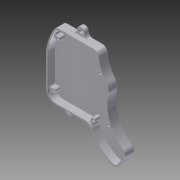
# Autodesk Inventor part: 20keyCaseRIght
Saved by Autodesk Inventor 2015 SP2 (Build 190223200, 223)
## iProperties
Created: 2015-12-14
Part Number: 20keyCaseRIght
Material: Aluminum 6061
Document SubType Name: Modeling
Designer: Josh
Density: 2.7 g/cm^3
Appearance: Aluminum - Flat
Author: Josh
Autodesk Inventor part; units mm, degrees
ref_plane "YZ Plane" through (0, 0, 0) normal (1, 0, 0) x (0, 1, 0)
ref_plane "XZ Plane" through (0, 0, 0) normal (0, 1, 0) x (-1, 0, 0)
ref_plane "XY Plane" through (0, 0, 0) normal (0, 0, 1) x (1, 0, 0)
sketch "Sketch1" plane through (0, 0, 0) normal (0, 0, 1) x (1, 0, 0)
  arc A0 (-34.3306, 52.1789) -> (-46.6208, 17.6368) centre (46.1813, 4.0752) ccw projected
  arc A1 (-46.6913, -8.336) -> (-46.6875, -8.1163) centre (-53.0375, -8.1163) ccw projected
  arc A2 (-46.6208, 17.6368) -> (-46.6875, 16.7186) centre (-40.3375, 16.7186) ccw projected
  arc A3 (-28.8795, 55.272) -> (-34.3306, 52.1789) centre (-28.8795, 48.922) ccw projected
  line L0 (-28.8795, 55.272) -> (26.3659, 55.272) projected
  arc A4 (32.6845, 49.5522) -> (26.3659, 55.272) centre (26.3659, 48.922) ccw projected
  arc A5 (32.6845, 49.5522) -> (45.4912, 18.6994) centre (90.0314, 55.272) ccw projected
  arc A6 (48.0197, 7.6526) -> (45.4912, 18.6994) centre (35.6761, 10.6401) ccw projected
  arc A7 (48.0197, 7.6526) -> (72.5516, -61.5815) centre (113.3553, -8.1601) ccw projected
  arc A8 (74.0573, -70.0323) -> (72.5516, -61.5815) centre (68.6971, -66.6278) ccw projected
  line L1 (65.6044, -83.341) -> (74.0573, -70.0323) projected
  arc A9 (58.0785, -85.9058) -> (65.6044, -83.341) centre (60.2442, -79.9365) ccw projected
  arc A10 (25.4201, -55.2506) -> (58.0785, -85.9058) centre (77.431, -32.5649) ccw projected
  arc A11 (25.4201, -55.2506) -> (13.7792, -47.628) centre (13.7792, -60.328) ccw projected
  arc A12 (-49.8625, -34.928) -> (-33.9875, -50.803) centre (-33.9875, -34.928) ccw
  arc A13 (-37.0562, 53.8074) -> (-49.7624, 18.0959) centre (46.1813, 4.0752) ccw
  arc A14 (-28.8795, 58.447) -> (-37.0562, 53.8074) centre (-28.8795, 48.922) ccw
  arc A15 (35.8439, 49.8674) -> (26.3659, 58.447) centre (26.3659, 48.922) ccw
  arc A16 (35.8439, 49.8674) -> (47.945, 20.7143) centre (90.0314, 55.272) ccw
  arc A17 (51.1056, 6.9058) -> (47.945, 20.7143) centre (35.6761, 10.6401) ccw
  arc A18 (51.1056, 6.9058) -> (74.4788, -59.0583) centre (113.3553, -8.1601) ccw
  arc A19 (76.7374, -71.7346) -> (74.4788, -59.0583) centre (68.6971, -66.6278) ccw
  arc A20 (22.5099, -56.5199) -> (13.7792, -50.803) centre (13.7792, -60.328) ccw
  line L2 (-33.9875, -34.928) -> (-33.9875, -63.8542)
  line L3 (-33.9875, -34.928) -> (-53.3277, -34.928)
  arc A21 (-49.7624, 18.0959) -> (-49.8625, 16.7186) centre (-40.3375, 16.7186) ccw
  line L4 (-40.3375, 16.7186) -> (-53.0375, 16.7186)
  line L5 (-40.3375, 16.7186) -> (-50.1751, 18.1562)
  line L6 (-28.8795, 48.922) -> (-38.906, 54.9127)
  line L7 (-28.8795, 48.922) -> (-28.8795, 65.0273)
  line L8 (26.3659, 48.922) -> (26.3659, 63.8949)
  line L9 (26.3659, 48.922) -> (41.6068, 50.4421)
  line L10 (35.6761, 10.6401) -> (50.953, 23.1841)
  line L11 (35.6761, 10.6401) -> (56.3542, 5.6355)
  line L12 (68.6971, -66.6278) -> (82.3318, -48.7769)
  line L13 (68.6971, -66.6278) -> (86.2238, -77.7598)
  line L14 (60.2442, -79.9365) -> (52.8937, -100.1965)
  line L15 (13.7792, -60.328) -> (13.7792, -43.3364)
  line L16 (13.7792, -60.328) -> (29.8025, -53.3391)
  line L17 (60.2442, -79.9365) -> (68.7206, -85.3202)
  arc A22 (56.9956, -88.8904) -> (68.2845, -85.0433) centre (60.2442, -79.9365) ccw
  arc A23 (22.5099, -56.5199) -> (56.9956, -88.8904) centre (77.431, -32.5649) ccw
  line L18 (68.2845, -85.0433) -> (76.7374, -71.7346)
  line L19 (-49.8625, -34.928) -> (-49.8625, 16.7186)
  line L20 (-33.9875, -50.803) -> (13.7792, -50.803)
  line L21 (-28.8795, 58.447) -> (26.3659, 58.447)
  circle A24 centre (12.1917, -49.2155) radius 1.5875
  line L22 (-46.6875, 16.7186) -> (-46.6875, -34.928) projected
  arc A25 (-46.6875, -34.928) -> (-33.9875, -47.628) centre (-33.9875, -34.928) ccw projected
  line L23 (13.7792, -47.628) -> (-33.9875, -47.628) projected
  point P0 (0, 0)
  point P1 (-33.9875, -51.1891)
  point P2 (-45.0507, -34.928)
  dimension "d0" = 3.175
  constraints: 40 end point, 32 point on line, 24 point on circle, 13 centre point, 12 concentric, 4 parallel, 3 tangent, 1 coincident, 1 midpoint
  measures "d0" diameter of A24
extrude "Extrusion1" add sketch "Sketch1" against normal blind 14.2875 contours L6 L7 L0 L8 L9 A5 L10 L11 A7 L12 L13 L1 L17 L14 A10 A11 L23 L2 L3 L22 L4 L5 A0 | L6 A14 L7 A3 | A3 L7 L6 | A0 L5 A13 L6 | L5 L4 A2 | A2 L4 A21 L5 | L7 L21 L8 L0 | L22 L3 L19 L4 | L8 A15 L9 A4 | A4 L9 L8 | L9 A16 L10 A5 | L3 A25 L2 A12 | L3 L2 A25 | L10 A17 L11 A6 | A6 L11 L10 | L2 L23 A24 L20 | L11 A18 L12 A7 | A24 L15 L20 | A24 | L23 L15 A24 | L12 A19 L13 A8 | A8 L13 L12 | L15 A11 L16 A20 | L13 L18 L17 L1 | L16 A10 L14 A23 | L17 A22 L14 A9 | A9 L14 L17
shell "Shell1" thickness 2.54 removed faces 1 at (4.4642, -12.5389, 0)
sketch "Sketch2" plane through (0, 0, -14.2875) normal (0, 0, -1) x (-1, 0, 0)
  arc A0 (7.6068, 64.797) -> (13.9568, 58.447) centre (13.9568, 64.797) ccw projected
  circle A1 centre (1.2568, 64.797) radius 6.35 projected
  circle A2 centre (1.2568, 64.797) radius 2.5527
  arc A3 (-11.4432, 58.447) -> (-5.0932, 64.797) centre (-11.4432, 64.797) ccw projected
  arc A4 (33.9875, -50.803) -> (27.6375, -57.153) centre (33.9875, -57.153) ccw projected
  circle A5 centre (21.2875, -57.153) radius 6.35 projected
  circle A6 centre (21.2875, -57.153) radius 2.5527
  arc A7 (14.9375, -57.153) -> (8.5875, -50.803) centre (8.5875, -57.153) ccw projected
  arc A8 (-25.6319, -62.6817) -> (-23.8454, -71.0319) centre (-20.1423, -65.8735) ccw projected
  circle A9 centre (-27.5485, -76.1904) radius 6.35 projected
  circle A10 centre (-27.5485, -76.1904) radius 2.5527
  arc A11 (-32.1676, -80.5477) -> (-40.6814, -79.8896) centre (-36.7867, -84.905) ccw projected
  arc A12 (-32.1676, -80.5477) -> (-40.6814, -79.8896) centre (-36.7867, -84.905) ccw
  arc A13 (-25.6319, -62.6817) -> (-23.8454, -71.0319) centre (-20.1423, -65.8735) ccw
  arc A14 (-56.9956, -88.8904) -> (-22.5099, -56.5199) centre (-77.431, -32.5649) ccw projected
  arc A15 (-23.8454, -71.0319) -> (-32.3284, -72.0101) centre (-27.5485, -76.1904) ccw
  arc A16 (-32.3284, -72.0101) -> (-32.1676, -80.5477) centre (-27.5485, -76.1904) ccw
  arc A17 (-40.6814, -79.8896) -> (-32.3284, -72.0101) centre (-77.431, -32.5649) ccw
  arc A18 (-32.3284, -72.0101) -> (-25.6319, -62.6817) centre (-77.431, -32.5649) ccw
  arc A19 (-56.9956, -88.8904) -> (-22.5099, -56.5199) centre (-77.431, -32.5649) ccw projected
  arc A20 (-11.4432, 58.447) -> (-5.0932, 64.797) centre (-11.4432, 64.797) ccw
  arc A21 (7.6068, 64.797) -> (13.9568, 58.447) centre (13.9568, 64.797) ccw
  arc A22 (1.2568, 58.447) -> (7.6068, 64.797) centre (1.2568, 64.797) ccw
  arc A23 (-5.0932, 64.797) -> (1.2568, 58.447) centre (1.2568, 64.797) ccw
  line L0 (-11.4432, 58.447) -> (1.2568, 58.447)
  line L1 (28.8795, 58.447) -> (-26.3659, 58.447) projected
  line L2 (1.2568, 58.447) -> (13.9568, 58.447)
  arc A24 (14.9375, -57.153) -> (8.5875, -50.803) centre (8.5875, -57.153) ccw
  arc A25 (33.9875, -50.803) -> (27.6375, -57.153) centre (33.9875, -57.153) ccw
  line L3 (-13.7792, -50.803) -> (33.9875, -50.803) projected
  arc A26 (27.6375, -57.153) -> (21.2875, -50.803) centre (21.2875, -57.153) ccw
  arc A27 (21.2875, -50.803) -> (14.9375, -57.153) centre (21.2875, -57.153) ccw
  line L4 (8.5875, -50.803) -> (21.2875, -50.803)
  line L5 (21.2875, -50.803) -> (33.9875, -50.803)
  circle A28 centre (1.2568, 64.797) radius 2.5527 projected
  circle A29 centre (21.2875, -57.153) radius 2.5527 projected
  circle A30 centre (-27.5485, -76.1904) radius 2.5527 projected
  point P0 (0, 0)
  constraints: 32 point on circle, 17 centre point, 11 equal radius, 9 tangent, 8 end point, 3 concentric, 2 collinear, 1 point on line
extrude "Extrusion2" add sketch "Sketch2" against normal blind 6.35
sketch "Sketch3" plane through (-28.8795, 55.907, -11.7475) normal (0, 0, 1) x (1, 0, 0)
  circle A0 centre (-5.3111, -15.386) radius 2.0828 projected
  circle A1 centre (-12.1636, -91.6238) radius 2.0828 projected
  circle A2 centre (51.9997, -100.6477) radius 2.0828 projected
  circle A3 centre (76.8372, -95.9142) radius 2.0828 projected
  circle A4 centre (62.894, -29.7847) radius 2.0828 projected
  line L0 (103.4728, -126.2798) -> (95.0198, -139.5885) projected
  arc A5 (86.7414, -142.4097) -> (95.0198, -139.5885) centre (89.1236, -135.8435) ccw projected
  arc A6 (53.7175, -111.4114) -> (86.7414, -142.4097) centre (106.3104, -88.4719) ccw projected
  arc A7 (53.7175, -111.4114) -> (42.6587, -104.17) centre (42.6587, -116.235) ccw projected
  line L1 (42.6587, -104.17) -> (-5.108, -104.17) projected
  arc A8 (-18.443, -90.835) -> (-5.108, -104.17) centre (-5.108, -90.835) ccw projected
  line L2 (-18.443, -90.835) -> (-18.443, -39.1884) projected
  arc A9 (-18.3696, -38.1784) -> (-18.443, -39.1884) centre (-11.458, -39.1884) ccw projected
  arc A10 (-5.9963, -3.4024) -> (-18.3696, -38.1784) centre (75.0607, -51.8319) ccw projected
  arc A11 (0, 0) -> (-5.9963, -3.4024) centre (0, -6.985) ccw projected
  line L3 (0, 0) -> (55.2453, 0) projected
  arc A12 (62.1959, -6.2918) -> (55.2453, 0) centre (55.2453, -6.985) ccw projected
  arc A13 (62.1959, -6.2918) -> (74.8615, -36.8046) centre (118.9109, -0.635) ccw projected
  arc A14 (77.5164, -48.4038) -> (74.8615, -36.8046) centre (64.5556, -45.2669) ccw projected
  arc A15 (77.5164, -48.4038) -> (101.8165, -116.9838) centre (142.2348, -64.0671) ccw projected
  arc A16 (103.4728, -126.2798) -> (101.8165, -116.9838) centre (97.5766, -122.5348) ccw projected
  line L4 (55.2453, 2.54) -> (0, 2.54) projected
  arc A17 (0, 2.54) -> (-8.1767, -2.0996) centre (0, -6.985) ccw projected
  arc A18 (-8.1767, -2.0996) -> (-20.8829, -37.8111) centre (75.0607, -51.8319) ccw projected
  arc A19 (-20.8829, -37.8111) -> (-20.983, -39.1884) centre (-11.458, -39.1884) ccw projected
  line L5 (-20.983, -39.1884) -> (-20.983, -90.835) projected
  arc A20 (-20.983, -90.835) -> (-5.108, -106.71) centre (-5.108, -90.835) ccw projected
  line L6 (-5.108, -106.71) -> (42.6587, -106.71) projected
  arc A21 (51.3893, -112.4269) -> (42.6587, -106.71) centre (42.6587, -116.235) ccw projected
  arc A22 (51.3893, -112.4269) -> (85.8751, -144.7974) centre (106.3104, -88.4719) ccw projected
  arc A23 (85.8751, -144.7974) -> (97.1639, -140.9503) centre (89.1236, -135.8435) ccw projected
  line L7 (97.1639, -140.9503) -> (105.6169, -127.6416) projected
  arc A24 (105.6169, -127.6416) -> (103.3583, -114.9653) centre (97.5766, -122.5348) ccw projected
  arc A25 (79.9851, -49.0012) -> (103.3583, -114.9653) centre (142.2348, -64.0671) ccw projected
  arc A26 (79.9851, -49.0012) -> (76.8245, -35.1927) centre (64.5556, -45.2669) ccw projected
  arc A27 (64.7233, -6.0397) -> (76.8245, -35.1927) centre (118.9109, -0.635) ccw projected
  arc A28 (64.7233, -6.0397) -> (55.2453, 2.54) centre (55.2453, -6.985) ccw projected
  circle A29 centre (-5.3111, -15.386) radius 3.175
  circle A30 centre (-12.1636, -91.6238) radius 3.175
  circle A31 centre (51.9997, -100.6477) radius 3.175
  circle A32 centre (76.8372, -95.9142) radius 3.175
  circle A33 centre (62.894, -29.7847) radius 3.175
  arc A34 (-18.443, -86.0844) -> (-13.7158, -88.8541) centre (-15.268, -86.0844) ccw
  arc A35 (-12.2517, -94.7976) -> (-14.5997, -100.2015) centre (-12.3397, -97.9714) ccw
  arc A36 (45.053, -104.41) -> (48.8414, -100.9729) centre (45.6831, -101.2981) ccw
  arc A37 (53.7175, -111.4114) -> (42.6587, -104.17) centre (42.6587, -116.235) ccw projected
  arc A38 (53.2022, -103.5862) -> (51.9576, -108.5477) centre (54.4046, -106.5247) ccw
  arc A39 (77.5164, -48.4038) -> (101.8165, -116.9838) centre (142.2348, -64.0671) ccw projected
  arc A40 (77.0716, -92.7479) -> (80.2611, -88.4203) centre (77.3061, -89.5815) ccw
  arc A41 (84.848, -97.8396) -> (79.4744, -97.6821) centre (82.1117, -99.4499) ccw
  arc A42 (63.062, -26.6142) -> (66.168, -22.2401) centre (63.2299, -23.4436) ccw
  arc A43 (70.9516, -31.4327) -> (65.587, -31.4665) centre (68.28, -33.1483) ccw
  arc A44 (-8.335, -7.5508) -> (-5.4209, -12.2129) centre (-5.5307, -9.0398) ccw
  arc A45 (-7.7704, -17.3941) -> (-13.1975, -18.2738) centre (-10.2297, -19.4022) ccw
  line L8 (-18.443, -90.835) -> (-18.443, -39.1884) projected
  arc A46 (-18.443, -90.835) -> (-5.108, -104.17) centre (-5.108, -90.835) ccw projected
  arc A47 (53.7175, -111.4114) -> (42.6587, -104.17) centre (42.6587, -116.235) ccw projected
  arc A48 (77.5164, -48.4038) -> (101.8165, -116.9838) centre (142.2348, -64.0671) ccw projected
  arc A49 (62.1959, -6.2918) -> (74.8615, -36.8046) centre (118.9109, -0.635) ccw projected
  arc A50 (-5.9963, -3.4024) -> (-18.3696, -38.1784) centre (75.0607, -51.8319) ccw projected
  point P0 (28.8795, -55.907)
  dimension "d6" = 6.35
  constraints: 42 point on circle, 20 tangent, 15 centre point, 14 equal radius, 5 coincident, 1 point on line
  measures "d6" diameter of A29
extrude "Extrusion3" add sketch "Sketch3" along normal blind 10.16 contours A41 A32 A40 A15 | A32 | A7 A36 A31 A38 | A31 | A43 A33 A42 A13 | A33 | A8 L2 A34 A30 A35 | A30 | A44 A29 A45 A10 | A29
thread "Thread1" size "8-32 UNC" class "2B" standard "ANSI Unified Screw Threads" full length
thread "Thread2" size "8-32 UNC" class "2B" standard "ANSI Unified Screw Threads" full length
thread "Thread3" size "8-32 UNC" class "2B" standard "ANSI Unified Screw Threads" full length
thread "Thread4" size "8-32 UNC" class "2B" standard "ANSI Unified Screw Threads" full length
thread "Thread5" size "8-32 UNC" class "2B" standard "ANSI Unified Screw Threads" full length
sketch "Sketch4" plane through (-49.8625, -34.928, 0) normal (-1, 0, 0) x (0, 0, 1)
  line L0 (-11.7475, -3.9626) -> (-11.7475, -9.3665) projected
  line L1 (-11.7475, -13.335) -> (-11.7475, -9.3665) projected
  line L2 (-11.7475, -13.575) -> (-11.7475, -13.335) projected
  line L3 (-11.7475, -13.575) -> (-11.7475, -10.1379) projected
  line L4 (-11.7475, -10.1379) -> (-11.7475, -12.7512) projected
  line L5 (-11.7475, -12.7512) -> (-11.7475, -17.7127) projected
  line L6 (-11.7475, -20.5764) -> (-11.7475, -17.7127) projected
  line L7 (-11.7475, -51.5747) -> (-11.7475, -20.5764) projected
  line L8 (-11.7475, -48.7535) -> (-11.7475, -51.5747) projected
  line L9 (-11.7475, -35.4448) -> (-11.7475, -48.7535) projected
  line L10 (-11.7475, -26.1488) -> (-11.7475, -35.4448) projected
  line L11 (-11.7475, -7.0046) -> (-11.7475, -26.1488) projected
  line L12 (-11.7475, -7.0046) -> (-11.7475, -6.8471) projected
  line L13 (-11.7475, -6.8471) -> (-11.7475, -1.9129) projected
  line L14 (-11.7475, -1.9129) -> (-11.7475, 2.4147) projected
  line L15 (-11.7475, 42.4312) -> (-11.7475, 2.4147) projected
  line L16 (-11.7475, 54.0304) -> (-11.7475, 42.4312) projected
  line L17 (-11.7475, 59.4023) -> (-11.7475, 54.0304) projected
  line L18 (-11.7475, 59.4023) -> (-11.7475, 59.3685) projected
  line L19 (-11.7475, 59.3685) -> (-11.7475, 64.2208) projected
  line L20 (-11.7475, 64.2208) -> (-11.7475, 68.5949) projected
  line L21 (-11.7475, 84.5432) -> (-11.7475, 68.5949) projected
  line L22 (-11.7475, 90.835) -> (-11.7475, 84.5432) projected
  line L23 (-11.7475, 87.4326) -> (-11.7475, 90.835) projected
  line L24 (-11.7475, 83.2842) -> (-11.7475, 87.4326) projected
  line L25 (-11.7475, 83.2842) -> (-11.7475, 78.6221) projected
  line L26 (-11.7475, 78.6221) -> (-11.7475, 73.4409) projected
  line L27 (-11.7475, 73.4409) -> (-11.7475, 72.5612) projected
  line L28 (-11.7475, 52.6566) -> (-11.7475, 72.5612) projected
  line L29 (-11.7475, 51.6466) -> (-11.7475, 52.6566) projected
  line L30 (-11.7475, 4.7506) -> (-11.7475, 51.6466) projected
  line L31 (-11.7475, 4.7506) -> (-11.7475, 1.9809) projected
  line L32 (-11.7475, 1.9809) -> (-11.7475, -3.9626) projected
  line L33 (-1.397, 26.7) -> (-1.397, 12.7) projected
  line L34 (0, 12.7) -> (0, 26.7) projected
  line L35 (0, 31.75) -> (0, 45.75) projected
  line L36 (-1.397, 45.75) -> (-1.397, 31.75) projected
  line L37 (-1.397, -17.7375) -> (-1.397, 65.21)
  line L38 (0, 26.7) -> (-1.397, 26.7)
  line L39 (-1.397, 26.7) -> (-1.397, 31.75)
  line L40 (-1.397, 31.75) -> (0, 31.75)
  line L41 (0, 31.75) -> (0, 26.7)
  line L42 (0, -6.35) -> (0, 7.65) projected
  line L43 (0, 7.65) -> (-1.397, 7.65)
  line L44 (-1.397, 7.65) -> (-1.397, 12.7)
  line L45 (-1.397, 12.7) -> (0, 12.7)
  line L46 (0, 12.7) -> (0, 7.65)
  line L47 (-1.397, 7.65) -> (-11.7475, 7.65)
  line L48 (-11.7475, 7.65) -> (-11.7475, 12.7)
  line L49 (-11.7475, 12.7) -> (-1.397, 12.7)
  line L50 (-1.397, 12.7) -> (-1.397, 7.65)
  line L51 (-1.397, 26.7) -> (-11.7475, 26.7)
  line L52 (-11.7475, 26.7) -> (-11.7475, 31.75)
  line L53 (-11.7475, 31.75) -> (-1.397, 31.75)
  line L54 (-1.397, 31.75) -> (-1.397, 26.7)
  line L55 (-11.7475, 7.65) -> (-1.397, 12.7)
  line L56 (-11.7475, 12.7) -> (-1.397, 7.65)
  line L57 (-11.7475, 26.7) -> (-1.397, 31.75)
  line L58 (-11.7475, 31.75) -> (-1.397, 26.7)
  circle A0 centre (-6.5722, 10.175) radius 4.0005
  line L59 (-2.7622, 24.4625) -> (-10.3822, 24.4625)
  line L60 (-10.3822, 24.4625) -> (-10.3822, 33.9875)
  line L61 (-10.3822, 33.9875) -> (-2.7622, 33.9875)
  line L62 (-2.7622, 33.9875) -> (-2.7622, 24.4625)
  line L63 (-2.7622, 24.4625) -> (-10.3822, 33.9875) construction
  line L64 (-10.3822, 24.4625) -> (-2.7622, 33.9875) construction
  arc A1 (-10.5184, 25.2563) -> (-8.1372, 22.875) centre (-8.1372, 25.2563) ccw
  arc A2 (-5.0073, 22.875) -> (-2.6261, 25.2563) centre (-5.0073, 25.2563) ccw
  arc A3 (-2.6261, 33.1938) -> (-5.0073, 35.575) centre (-5.0073, 33.1938) ccw
  arc A4 (-8.1372, 35.575) -> (-10.5184, 33.1938) centre (-8.1372, 33.1938) ccw
  line L65 (-10.5184, 25.2563) -> (-10.5184, 33.1938)
  line L66 (-8.1372, 22.875) -> (-5.0073, 22.875)
  line L67 (-2.6261, 25.2563) -> (-2.6261, 33.1938)
  line L68 (-5.0073, 35.575) -> (-8.1372, 35.575)
  line L69 (0, 22.875) -> (-5.2816, 22.875)
  line L70 (-5.2816, 22.875) -> (-5.2816, 35.575)
  line L71 (-5.2816, 35.575) -> (0, 35.575)
  line L72 (0, 35.575) -> (0, 22.875)
  line L73 (0, 22.875) -> (-0.6985, 22.875)
  line L74 (-0.6985, 22.875) -> (-0.6985, 26.7)
  line L75 (-0.6985, 26.7) -> (0, 26.7)
  line L76 (0, 26.7) -> (0, 22.875)
  line L77 (-0.6985, 31.75) -> (0, 31.75)
  line L78 (0, 31.75) -> (0, 35.575)
  line L79 (0, 35.575) -> (-0.6985, 35.575)
  line L80 (-0.6985, 35.575) -> (-0.6985, 31.75)
  point P0 (0, 34.928)
  point P1 (-6.5722, 29.225)
  dimension "d19" = 8.001
  dimension "d20" = 9.525
  dimension "d21" = 7.62
  dimension "d22" = 2.3813
  dimension "d23" = 12.7
  constraints: 86 end point, 21 parallel, 12 point on circle, 9 horizontal, 8 perpendicular, 8 tangent, 6 midpoint, 5 centre point, 5 point on line, 4 collinear, 3 equal radius
  measures "d19" diameter of A0
  measures "d20" distance of L59.end L60.end
  measures "d21" distance of L60.end L61.end
  measures "d22" radius of A1
  measures "d23" distance of L69.end L70.end
extrude "Extrusion4" cut sketch "Sketch4" against normal blind 8.763 contours L65 A4 L60 L53 | L53 L60 L58 L65 | L58 L60 L57 L65 | L65 L57 L60 L51 | L51 L60 A1 L65 | L60 L61 L70 L53 | L53 L70 L57 L58 L60 | L58 L57 L60 | A0 L49 | L49 A0 L55 L56 | L56 L55 A0 | L60 L57 L58 L70 L51 | L51 L70 L59 L60 | L70 L61 L62 L53 | L53 L62 L57 L70 | A4 L68 L70 L61 | L57 L70 L58 | A0 L55 L56 L47 | L47 A0 | L55 A0 L56 | L70 L58 L62 L51 | L51 L62 L59 L70 | L59 L70 L66 A1 | L62 A3 L67 L53 | L53 L67 L57 L62 | L57 L62 L58 L70 | L70 L68 A3 L61 | L62 L58 L67 L51 | L51 L67 A2 L62 | L59 A2 L66 L70 | L57 L67 L58 L62
body "Solid1"
